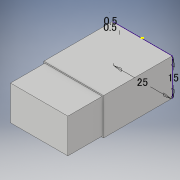
# Autodesk Inventor part: eraser
Saved by Autodesk Inventor 2019 (Build 230136000, 136)
## iProperties
Created: 2020-11-03
Part Number: eraser
Material: 一般
Document SubType Name: Modeling
Designer: masato
Density: 1 g/cm^3
Appearance: 既定
Author: masato
## iProperties of the stored document eraser_3D プリント.ipt
Created: 2020-11-03
Part Number: eraser_3D プリント
Material: 一般
Document SubType Name: Modeling
Designer: masato
Density: 1 g/cm^3
Appearance: 既定
Author: masato
Autodesk Inventor part; units mm, degrees
ref_plane "YZ Plane" through (0, 0, 0) normal (1, 0, 0) x (0, 1, 0)
ref_plane "XZ Plane" through (0, 0, 0) normal (0, 1, 0) x (-1, 0, 0)
ref_plane "XY Plane" through (0, 0, 0) normal (0, 0, 1) x (1, 0, 0)
sketch "スケッチ1" plane through (0, 0, 0) normal (0, 0, 1) x (1, 0, 0)
  line L0 (-12.5, 7.5) -> (12.5, 7.5)
  line L1 (12.5, 7.5) -> (12.5, -7.5)
  line L2 (12.5, -7.5) -> (-12.5, -7.5)
  line L3 (-12.5, -7.5) -> (-12.5, 7.5)
  line L4 (-12.5, 7.5) -> (12.5, -7.5) construction
  line L5 (12.5, 7.5) -> (-12.5, -7.5) construction
  line L6 (-13, 8) -> (13, 8)
  line L7 (13, 8) -> (13, -8)
  line L8 (13, -8) -> (-13, -8)
  line L9 (-13, -8) -> (-13, 8)
  line L10 (-13, 8) -> (13, -8) construction
  line L11 (13, 8) -> (-13, -8) construction
  point P0 (0, 0)
  dimension "d0" = 25
  dimension "d1" = 15
  dimension "d4" = 0.5
  dimension "d5" = 0.5
  constraints: 24 end point, 4 midpoint, 4 parallel, 2 horizontal, 2 perpendicular
  measures "d0" distance of L1.end L2.end
  measures "d1" distance of L0.end L1.end
  measures "d4" distance between parallel lines of L6 L0
  measures "d5" distance between parallel lines of L3 L9
extrude "押し出し1" add sketch "スケッチ1" along normal blind 45 contours L0 L1 L2 L3
extrude "押し出し2" add sketch "スケッチ1" along normal blind 30
sketch "スケッチ2" plane through (-13, 8, 0) normal (0, 1, 0) x (1, 0, 0)
  point P0 (13, 0)
